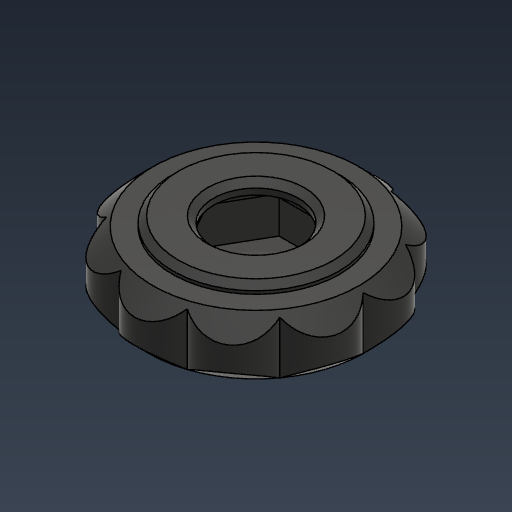
# Autodesk Inventor part: Raendelmutter M4 Druckteil
Saved by Autodesk Inventor 2023.1 (Build 271208000, 208)
## iProperties
Part Number: Raendelmutter M4 Druckteil
Material: PC/ABS-Kunststoff
Document SubType Name: Modeling
Designer: rYan
Density: 0.357273 g/cm^3
Appearance: Glatt - Schwarz
Mass: 0.213031 g
Surface Area: 6.65478 cm^2
Volume: 0.59627 cm^3
Author: rYan
Autodesk Inventor part; units mm, degrees
ref_plane "YZ Plane" through (0, 0, 0) normal (1, 0, 0) x (0, 1, 0)
ref_plane "XZ Plane" through (0, 0, 0) normal (0, 1, 0) x (-1, 0, 0)
ref_plane "XY Plane" through (0, 0, 0) normal (0, 0, 1) x (1, 0, 0)
sketch "Skizze1" plane through (0, 0, 0) normal (0, 0, 1) x (1, 0, 0)
  circle A0 centre (0, 0) radius 8 construction
  arc A1 (2.183, 6.7185) -> (-2.183, 6.7185) centre (0, 5.5) ccw
  line L0 (0, 11.2) -> (0, -11.2) projected
  line L1 (-2.183, 6.7185) -> (2.183, 6.7185) construction
  line L2 (-2.183, 6.7185) -> (0, 0)
  line L3 (0, 0) -> (2.183, 6.7185)
  dimension "d0" = 16
  dimension "d2" = 36
  dimension "d31" = 2.5
  constraints: 6 end point, 2 centre point, 2 point on circle, 1 coincident, 1 horizontal, 1 point on line, 1 tangent
  measures "d0" diameter of A0
  measures "d2" angle of L2 L3
  measures "d31" radius of A1
extrude "Extrusion1" add sketch "Skizze1" along normal blind 4
pattern_circular "Runde Anordnung1" count 10 over 360 about axis through (0, 0, -10) along (0, 0, 1) of "Extrusion1"
sketch "Skizze2" plane through (0, 0, 4) normal (0, 0, 1) x (1, 0, 0)
  line L0 (0, 11.2) -> (0, -11.2) projected
  line L1 (2.0785, 3.6) -> (4.1569, 0)
  line L2 (4.1569, 0) -> (2.0785, -3.6)
  line L3 (2.0785, -3.6) -> (-2.0785, -3.6)
  line L4 (-2.0785, -3.6) -> (-4.1569, 0)
  line L5 (-4.1569, 0) -> (-2.0785, 3.6)
  line L6 (-2.0785, 3.6) -> (2.0785, 3.6)
  point P0 (0, 0)
  point P1 (0, 0)
  point P2 (0, 3.6)
  dimension "d8" = 7.2
  constraints: 12 end point, 1 coincident, 1 midpoint, 1 point on line, 13 other
  measures "d8" distance between parallel lines of L3 L6
extrude "Extrusion2" cut sketch "Skizze2" against normal blind 3.4
sketch "Skizze3" plane through (0, 0, 4) normal (0, 0, 1) x (1, 0, 0)
  circle A0 centre (0, 0) radius 5.5
  circle A1 centre (0, 0) radius 2.8
  dimension "d11" = 11
  dimension "d14" = 5.6
  constraints: 2 centre point, 2 coincident
  measures "d11" diameter of A0
  measures "d14" diameter of A1
extrude "Extrusion3" add sketch "Skizze3" along normal blind 0.6 and the other way blind 0.2
chamfer "Fase1" distance 0.4 angle 45 1 edges at (-5.5, 0, 4.6)
sketch "Skizze4" plane through (0, 0, 0) normal (0, 1, 0) x (-1, 0, 0)
  line L0 (0, 0) -> (0, 7.735)
  line L1 (-8, 1.2) -> (-6.8, 0)
  line L2 (-8, 1.2) -> (-8, 2.8)
  line L3 (-6.8, 4) -> (-8, 2.8)
  line L4 (-6.8, 0) -> (-8.9431, 0)
  line L5 (-8.9431, 0) -> (-8.9431, 4)
  line L6 (-8.9431, 4) -> (-6.8, 4)
  line L7 (-8, 2) -> (0, 2) construction
  line L8 (-5.5, 4) -> (5.5, 4) projected
  line L9 (-2.183, 4) -> (2.183, 4) projected
  line L10 (2.183, 4) -> (5.7151, 4) projected
  line L11 (5.7151, 4) -> (7.0642, 4) projected
  line L12 (7.0642, 4) -> (5.7151, 4) projected
  line L13 (5.7151, 4) -> (2.183, 4) projected
  line L14 (2.183, 4) -> (-2.183, 4) projected
  line L15 (-2.183, 4) -> (-5.7151, 4) projected
  line L16 (-5.7151, 4) -> (-7.0642, 4) projected
  line L17 (-7.0642, 4) -> (-5.7151, 4) projected
  line L18 (-5.7151, 4) -> (-2.183, 4) projected
  line L19 (2.183, 0) -> (-2.183, 0) projected
  line L20 (-2.183, 0) -> (-5.7151, 0) projected
  line L21 (-5.7151, 0) -> (-7.0642, 0) projected
  line L22 (-7.0642, 0) -> (-5.7151, 0) projected
  line L23 (-5.7151, 0) -> (-2.183, 0) projected
  line L24 (-2.183, 0) -> (2.183, 0) projected
  line L25 (2.183, 0) -> (5.7151, 0) projected
  line L26 (5.7151, 0) -> (7.0642, 0) projected
  line L27 (7.0642, 0) -> (5.7151, 0) projected
  line L28 (5.7151, 0) -> (2.183, 0) projected
  dimension "d18" = 1.6
  dimension "d19" = 45
  dimension "d25" = 16
  constraints: 16 end point, 3 perpendicular, 3 point on line, 1 coincident, 1 horizontal, 1 midpoint, 1 symmetric about line, 1 vertical, 1 other
  measures "d18" distance of L2.end L1.start
  measures "d19" angle of L4 L1
  measures "d25" diameter of L2 L0
revolve "Umdrehung1" cut sketch "Skizze4" angle 360 about axis through (0, 0, 0) along (0, 0, 1) contours L4 L5 L6 L3 L2 L1
chamfer "Fase2" distance 0.4 angle 45 1 edges at (-2.8, 0, 4.6)
fillet "Rundung1" radius 1 1 edges at (-6.8, 0, 0)
sketch "Skizze5" plane through (0, 0, 3.8) normal (0, 0, -1) x (-1, 0, 0)
  circle A0 centre (0, 0) radius 2.8 projected
  line L0 (2.0785, 3.6) -> (4.1569, 0) projected
  line L1 (-2.0785, 3.6) -> (2.0785, 3.6) projected
  line L2 (-4.1569, 0) -> (-2.0785, 3.6) projected
  line L3 (-2.0785, -3.6) -> (-4.1569, 0) projected
  line L4 (2.0785, -3.6) -> (-2.0785, -3.6) projected
  line L5 (4.1569, 0) -> (2.0785, -3.6) projected
  line L6 (-3.2332, 0) -> (-1.6166, 2.8)
  line L7 (-1.6166, 2.8) -> (1.6166, 2.8)
  line L8 (1.6166, 2.8) -> (3.2332, 0)
  line L9 (3.2332, 0) -> (1.6166, -2.8)
  line L10 (1.6166, -2.8) -> (-1.6166, -2.8)
  line L11 (-1.6166, -2.8) -> (-3.2332, 0)
  constraints: 12 end point, 1 tangent, 5 other
extrude "Extrusion4" add sketch "Skizze5" along normal blind 0.2
